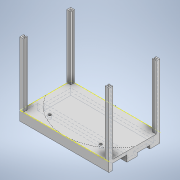
# Autodesk Inventor part: NL housing_Main
Saved by Autodesk Inventor 2022 (Build 260153000, 153)
## iProperties
Created: 2021-09-23
Part Number: NL housing_Main
Material: Generic
Document SubType Name: Modeling
Designer: andri
Density: 1 g/cm^3
Appearance: Default
Author: andri
Autodesk Inventor part; units mm, degrees
ref_plane "YZ Plane" through (0, 0, 0) normal (1, 0, 0) x (0, 1, 0)
ref_plane "XZ Plane" through (0, 0, 0) normal (0, 1, 0) x (-1, 0, 0)
ref_plane "XY Plane" through (0, 0, 0) normal (0, 0, 1) x (1, 0, 0)
sketch "Sketch1" plane through (0, 0, 0) normal (0, 1, 0) x (-1, 0, 0)
  line L0 (0, 0) -> (140, 0)
  line L1 (140, 0) -> (140, 80)
  line L2 (140, 80) -> (0, 80)
  line L3 (0, 80) -> (0, 0)
  dimension "d0" = 140
  dimension "d1" = 80
  constraints: 8 end point, 2 parallel, 1 horizontal, 1 perpendicular
  measures "d0" distance of L1.end L2.end
  measures "d1" distance between parallel lines of L0 L2
extrude "Extrusion2" add sketch "Sketch1" against normal blind 15
sketch "Sketch2" plane through (0, 0, 80) normal (1, 0, 0) x (0, 0, -1)
  line L0 (0, -15) -> (80, -15) projected
  line L1 (5, -5) -> (28.1523, -5)
  line L2 (28.1523, -5) -> (28.1523, -15)
  line L3 (5, -5) -> (5, -15)
  line L4 (80, 0) -> (80, -15) projected
  line L5 (0, 0) -> (0, -15) projected
  line L6 (0, 0) -> (80, 0) projected
  dimension "d6" = 5
  dimension "d7" = 5
  dimension "d8" = 51.8477
  constraints: 6 end point, 2 point on line, 1 horizontal, 1 parallel, 1 perpendicular
  measures "d6" distance between parallel lines of L5 L3
  measures "d7" distance between parallel lines of L6 L1
  measures "d8" distance between parallel lines of L4 L2
extrude "Extrusion3" cut sketch "Sketch2" against normal through all contours L3 L1 L2 L0
sketch "Sketch3" plane through (0, -15, 0) normal (0, -1, 0) x (1, 0, 0)
  line L0 (0, 51.8477) -> (-140, 51.8477) projected
  line L1 (-140, 51.8477) -> (-140, 0) projected
  line L2 (-140, 0) -> (0, 0) projected
  line L3 (0, 0) -> (0, 51.8477) projected
  line L4 (-5, 5) -> (-135, 5)
  line L5 (-135, 5) -> (-135, 46.8477)
  line L6 (-135, 46.8477) -> (-5, 46.8477)
  line L7 (-5, 46.8477) -> (-5, 5)
  dimension "d11" = 5
  constraints: 8 end point, 3 other
  measures "d11" distance between parallel lines of L4 L2
extrude "Electronics_Housing" cut sketch "Sketch3" against normal blind 10 contours L4 L5 L6 L7
sketch "Sketch4" plane through (0, 0, 0) normal (0, 1, 0) x (1, 0, 0)
  circle A0 centre (-110, -63.0196) radius 2
  line L0 (0, 0) -> (-140, 0) projected
  line L1 (-70, 0) -> (-70, -80) construction
  line L2 (0, -80) -> (-140, -80) projected
  circle A1 centre (-30, -63.0196) radius 2
  dimension "d14" = 40
  dimension "d15" = 4
  constraints: 2 centre point, 2 end point, 2 midpoint, 1 symmetric about line, 1 other
  measures "d14" distance from line of L1 A0.centre
  measures "d15" diameter of A0
extrude "M4_Litho_Holder" cut sketch "Sketch4" against normal through all
sketch "Litho_Dimension" plane through (0, 0, 0) normal (0, 1, 0) x (1, 0, 0)
  line L0 (0, 0) -> (-140, 0) projected
  line L1 (-140, 0) -> (-140, -80) projected
  arc A0 (-140, -38.7298) -> (0.3875, -38.0211) centre (-70, 0) ccw construction
  line L2 (-140, -80) -> (0, -80) projected
  constraints: 2 point on circle, 1 centre point, 1 midpoint, 1 point on line, 1 tangent
sketch "Sketch6" plane through (0, -15, 0) normal (0, -1, 0) x (1, 0, 0)
  line L0 (0, 80) -> (0, 0) projected
  line L1 (-5, 46.8477) -> (-5, 5) projected
  line L2 (0, 15.9239) -> (-5, 15.9239)
  line L3 (-5, 15.9239) -> (-5, 35.9239)
  line L4 (-5, 35.9239) -> (0, 35.9239)
  line L5 (0, 35.9239) -> (0, 15.9239)
  line L6 (-140, 0) -> (0, 0) projected
  line L7 (0, 51.8477) -> (-140, 51.8477) projected
  point P0 (0, 35.9239)
  dimension "d18" = 15.9238
  dimension "d19" = 20
  dimension "d20" = 15.9238
  constraints: 8 end point, 2 parallel, 2 point on line, 1 horizontal, 1 perpendicular
  measures "d18" distance between parallel lines of L2 L6
  measures "d19" distance between parallel lines of L4 L2
  measures "d20" distance between parallel lines of L7 L4
extrude "ARd_Nano_Mount" cut sketch "Sketch6" against normal blind 5
sketch "Sketch7" plane through (0, 0, 0) normal (0, 1, 0) x (1, 0, 0)
  line L0 (-140, -80) -> (0, -80) construction
  line L1 (-140, -80) -> (-134, -80)
  line L2 (-134, -80) -> (-134, -74)
  line L3 (-134, -74) -> (-140, -74)
  line L4 (-140, -74) -> (-140, -80)
  line L5 (-140, 0) -> (-140, -80) projected
  line L6 (0, -80) -> (0, 0) projected
  line L7 (-138, -74) -> (-138, -78)
  line L8 (-138, -78) -> (-134, -78)
  line L9 (-136, -74) -> (-136, -76)
  line L10 (-136, -76) -> (-134, -76)
  line L11 (-70, -80) -> (-70, 0) construction
  line L12 (0, 0) -> (-140, 0) projected
  line L13 (-140, -40) -> (0, -40) construction
  line L14 (0, -80) -> (-6, -80)
  line L15 (-6, -80) -> (-6, -74)
  line L16 (-6, -74) -> (0, -74)
  line L17 (0, -74) -> (0, -80)
  line L18 (-2, -74) -> (-2, -78)
  line L19 (-2, -78) -> (-6, -78)
  line L20 (-4, -74) -> (-4, -76)
  line L21 (-4, -76) -> (-6, -76)
  line L22 (-140, 0) -> (-134, 0)
  line L23 (-134, 0) -> (-134, -6)
  line L24 (-134, -6) -> (-140, -6)
  line L25 (-140, -6) -> (-140, 0)
  line L26 (-138, -6) -> (-138, -2)
  line L27 (-138, -2) -> (-134, -2)
  line L28 (-136, -6) -> (-136, -4)
  line L29 (-136, -4) -> (-134, -4)
  line L30 (-6, 0) -> (-6, -6)
  line L31 (-4, -6) -> (-4, -4)
  line L32 (-4, -4) -> (-6, -4)
  line L33 (-2, -6) -> (-2, -2)
  line L34 (0, 0) -> (-6, 0)
  line L35 (-6, -6) -> (0, -6)
  line L36 (0, -6) -> (0, 0)
  line L37 (-2, -2) -> (-6, -2)
  point P0 (0, -6)
  dimension "d27" = 2
  dimension "d29" = 2
  dimension "d30" = 2
  constraints: 68 end point, 27 symmetric about line, 10 point on line, 6 perpendicular, 4 midpoint, 2 parallel, 1 horizontal, 1 vertical, 1 other
  measures "d27" distance between parallel lines of L4 L7
  measures "d29" distance between parallel lines of L7 L9
  measures "d30" distance between parallel lines of L2 L9
extrude "Extrusion7" add sketch "Sketch7" along normal blind 99.7 contours L4 L3 L7 L8 L2 L1 | L6 L14 L15 L19 L18 L16 | L12 L6 L35 L33 L37 L30 | L5 L12 L23 L27 L26 L24 | L10 L9 L3 L2 | L28 L29 L23 L24 | L32 L31 L35 L30 | L20 L21 L15 L16
equation "\"d18\" = d20"
body "Solid2"
